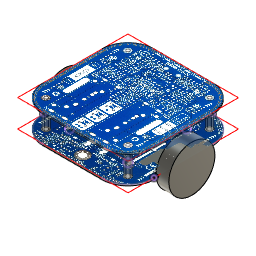
NIBO-Burger_Tuning (Autodesk Fusion 360 design; units mm, degrees)
Autodesk Fusion 360 part; units mm, degrees
sketch "Sketch1" plane through (0, 0, 0) normal (0, 0, 1) x (1, 0, 0) in component "Nibo Burger PCB Bottom"
  line L0 (25.4, 0) -> (82.6, 0)
  line L1 (108, 25.4) -> (108, 82.6)
  line L2 (82.6, 108) -> (25.4, 108)
  line L3 (0, 82.6) -> (0, 25.4)
  arc A0 (25.4, 108) -> (0, 82.6) centre (25.4, 82.6) ccw
  arc A1 (108, 82.6) -> (82.6, 108) centre (82.6, 82.6) ccw
  arc A2 (82.6, 0) -> (108, 25.4) centre (82.6, 25.4) ccw
  arc A3 (0, 25.4) -> (25.4, 0) centre (25.4, 25.4) ccw
  point P0 (108, 0)
  point P1 (0, 108)
  dimension "d1" = 108
  dimension "d2" = 108
  dimension "d5" = 25.4
  constraint horizontal L0
  constraint vertical L1
  constraint horizontal L2
  constraint vertical L3
  constraint coincident P1 L3
  constraint coincident P1 L2
  constraint tangent L3 A0
  constraint tangent L2 A0
  constraint tangent L2 A1
  constraint tangent L1 A1
  constraint equal A0 A1
  constraint coincident P0 L1
  constraint coincident P0 L0
  constraint tangent L1 A2
  constraint tangent L0 A2
  constraint equal A0 A2
  constraint coincident origin L0
  constraint coincident origin L3
  constraint tangent L0 A3
  constraint tangent L3 A3
  constraint equal A0 A3
  measures "d1" distance of origin P0
  measures "d2" distance of origin P1
  measures "d5" radius of A0
extrude "Extrude1" add sketch "Sketch1" along normal blind 1.6 makes body 1 in component "Nibo Burger PCB Bottom"
sketch "Sketch2" plane through (0, 0, 1.6) normal (0, 0, 1) x (-1, 0, 0)
  line L0 (0, -82.6) -> (0, -25.4)
  line L1 (-25.4, 0) -> (-82.6, 0)
  line L2 (-108, -25.4) -> (-108, -82.6)
  line L3 (-82.6, -108) -> (-25.4, -108)
  arc A0 (0, -25.4) -> (-25.4, 0) centre (-25.4, -25.4) ccw
  arc A1 (-82.6, 0) -> (-108, -25.4) centre (-82.6, -25.4) ccw
  arc A2 (-108, -82.6) -> (-82.6, -108) centre (-82.6, -82.6) ccw
  arc A3 (-25.4, -108) -> (0, -82.6) centre (-25.4, -82.6) ccw
copy_body "CopyPasteBodies1" bodies 1 makes body 2 in component "Nibo Burger PCB Bottom"
move_body "Move1" bodies 2 to x (1, 0, 0) y (0, 1, 0) z (0, 0, 1) at (0, 0, 26.5) in component "Nibo Burger PCB Bottom"
copy_body "CutPasteBodies1" bodies 2 removing the originals makes body 3 in component "Nibo Burger PCB Top"
sketch "Sketch1 (2)" plane through (0, 0, 28.1) normal (0, 0, 1) x (-1, 0, 0) in component "Nibo Burger PCB Top"
  arc A0 (0, -25.4) -> (-25.4, 0) centre (-25.4, -25.4) ccw
  line L0 (-25.4, 0) -> (-82.6, 0)
  arc A1 (-82.6, 0) -> (-108, -25.4) centre (-82.6, -25.4) ccw
  line L1 (-108, -25.4) -> (-108, -82.6)
  arc A2 (-108, -82.6) -> (-82.6, -108) centre (-82.6, -82.6) ccw
  line L2 (-82.6, -108) -> (-25.4, -108)
  arc A3 (-25.4, -108) -> (0, -82.6) centre (-25.4, -82.6) ccw
  line L3 (0, -82.6) -> (0, -25.4)
  line L4 (0, -54) -> (-108, -54)
  line L5 (-94, -14) -> (-14, -14)
  line L6 (-14, -14) -> (-14, -94)
  line L7 (-14, -94) -> (-94, -94)
  line L8 (-94, -94) -> (-94, -14)
  line L9 (-94, -14) -> (-14, -94) construction
  line L10 (-14, -14) -> (-94, -94) construction
  point P0 (-54, -54)
  dimension "d7" = 80
  dimension "d8" = 80
  constraint midpoint L3 L4.start
  constraint midpoint L1 L4.end
  constraint horizontal L5
  constraint perpendicular L5 L6
  constraint parallel L5 L7
  constraint parallel L6 L8
  constraint coincident L9 P0
  constraint coincident L10 P0
  constraint midpoint L4 P0
  measures "d7" distance of L6.end L7.end
  measures "d8" distance of L5.end L6.end
hole "Hole1" at (14, 94, 28.1) at (94, 94, 28.1) at (14, 14, 28.1) at (94, 14, 28.1) direction (0, 0, -1) diameter 3.3 depth 30 tip angle 118 bodies 1 in component "Nibo Burger PCB Bottom"
hole "Hole1'" at (14, 94, 28.1) at (94, 94, 28.1) at (14, 14, 28.1) at (94, 14, 28.1) direction (0, 0, -1) diameter 3.3 depth 30 tip angle 118 bodies 3 in component "Nibo Burger PCB Top"
sketch "Sketch2 (2)" plane through (0, 0, 1.6) normal (0, 0, 1) x (-1, 0, 0) in component "Nibo Burger PCB Bottom"
  line L0 (-91.2116, -14.7471) -> (-91.9588, -11.9588)
  line L1 (-91.9588, -11.9588) -> (-94.7471, -11.2116)
  line L2 (-94.7471, -11.2116) -> (-96.7884, -13.2529)
  line L3 (-96.7884, -13.2529) -> (-96.0412, -16.0412)
  line L4 (-96.0412, -16.0412) -> (-93.2529, -16.7884)
  line L5 (-93.2529, -16.7884) -> (-91.2116, -14.7471)
  line L6 (-11.1966, -14.6888) -> (-12.0018, -11.9166)
  line L7 (-12.0018, -11.9166) -> (-14.8052, -11.2278)
  line L8 (-14.8052, -11.2278) -> (-16.8034, -13.3112)
  line L9 (-16.8034, -13.3112) -> (-15.9982, -16.0834)
  line L10 (-15.9982, -16.0834) -> (-13.1948, -16.7722)
  line L11 (-13.1948, -16.7722) -> (-11.1966, -14.6888)
  line L12 (-16.5376, -92.6238) -> (-16.4606, -95.5095)
  line L13 (-16.4606, -95.5095) -> (-13.9231, -96.8857)
  line L14 (-13.9231, -96.8857) -> (-11.4624, -95.3762)
  line L15 (-11.4624, -95.3762) -> (-11.5394, -92.4905)
  line L16 (-11.5394, -92.4905) -> (-14.0769, -91.1143)
  line L17 (-14.0769, -91.1143) -> (-16.5376, -92.6238)
  line L18 (-96.6547, -92.866) -> (-96.3094, -95.7321)
  line L19 (-96.3094, -95.7321) -> (-93.6547, -96.866)
  line L20 (-93.6547, -96.866) -> (-91.3453, -95.134)
  line L21 (-91.3453, -95.134) -> (-91.6906, -92.268)
  line L22 (-91.6906, -92.268) -> (-94.3453, -91.134)
  line L23 (-94.3453, -91.134) -> (-96.6547, -92.866)
  point P0 (-94, -14)
  point P1 (-14, -14)
  point P2 (-14, -94)
  point P3 (-94, -94)
  dimension "d15" = 2.5
  dimension "d16" = 2.5
  dimension "d17" = 2.5
  dimension "d18" = 2.5
  measures "d15" distance of P0 L5
  measures "d16" distance of P1 L11
  measures "d17" distance of P2 L17
  measures "d18" distance of P3 L23
extrude "Extrude2" add sketch "Sketch2 (2)" along normal blind 25 separate body makes body 4 at (14.8972, 91.6174, 9.9333) makes body 5 at (91.4607, 13.8177, 9.9333) makes body 6 at (16.535, 14.2353, 9.9333) makes body 7 at (91.4604, 94.1786, 9.9333) in component "Nibo Burger PCB Bottom"
sketch "Sketch3" plane through (0, 0, 1.6) normal (0, 0, 1) x (-1, 0, 0) in component "Nibo Burger PCB Bottom"
  line L0 (0, 0) -> (0, -54)
  line L1 (0, -54) -> (-108, -54)
  line L2 (-5.5, -78) -> (5.5, -78)
  line L3 (5.5, -78) -> (5.5, -30)
  line L4 (5.5, -30) -> (-5.5, -30)
  line L5 (-5.5, -30) -> (-5.5, -78)
  line L6 (-5.5, -78) -> (5.5, -30) construction
  line L7 (5.5, -78) -> (-5.5, -30) construction
  line L8 (-102.5, -78) -> (-113.5, -78)
  line L9 (-113.5, -78) -> (-113.5, -30)
  line L10 (-113.5, -30) -> (-102.5, -30)
  line L11 (-102.5, -30) -> (-102.5, -78)
  line L12 (-102.5, -78) -> (-113.5, -30) construction
  line L13 (-113.5, -78) -> (-102.5, -30) construction
  point P0 (0, -54)
  point P1 (-108, -54)
  dimension "d22" = 54
  dimension "d23" = 108
  dimension "d24" = 11
  dimension "d25" = 48
  dimension "d26" = 11
  dimension "d27" = 48
  constraint coincident L0.start origin
  constraint vertical L0
  constraint perpendicular L0 L1
  constraint horizontal L2
  constraint perpendicular L2 L3
  constraint parallel L2 L4
  constraint parallel L3 L5
  constraint coincident L6 P0
  constraint coincident L7 P0
  constraint coincident P0 L0.end
  constraint horizontal L8
  constraint perpendicular L8 L9
  constraint parallel L8 L10
  constraint parallel L9 L11
  constraint coincident L12 P1
  constraint coincident L13 P1
  constraint coincident P1 L1.end
  measures "d22" distance of L0.start P0
  measures "d23" distance of P0 P1
  measures "d24" distance of L3.end L4.end
  measures "d25" distance of L2.end L3.end
  measures "d26" distance of L9.end L10.end
  measures "d27" distance of L8.end L9.end
extrude "Extrude3" cut sketch "Sketch3" against normal blind 10 bodies 1 in component "Nibo Burger PCB Bottom"
sketch "Sketch4" plane through (0, 0, 0) normal (-1, 0, 0) x (0, -1, 0) in component "Nibo Burger PCB Bottom"
  line L0 (-78, 0) -> (-78, 1.6)
  line L1 (-78, 1.6) -> (-82.6, 1.6)
  line L2 (-82.6, 1.6) -> (-82.6, 0)
  line L3 (-82.6, 0) -> (-78, 0)
  line L4 (-78, 1.6) -> (-30, 1.6)
  circle A0 centre (-54, -0.7) radius 22.5
  circle A1 through (-31.5, -0.7, -108) (-65.25, 18.7856, -108) (-65.25, -20.1856, -108)
  dimension "d30" = 45
  dimension "d31" = 45
  constraint coincident L0.end L1.start
  constraint perpendicular L0 L4
  measures "d30" diameter of A0
extrude "Extrude4" add sketch "Sketch4" along normal blind 8.5 separate body contours L4 A0 | L4 A0 makes body 8 in component "Nibo Burger PCB Bottom"
extrude "Extrude5" add sketch "Sketch4" against normal blind 8.5 separate body contours A1 in plane through (108, 0, 0) normal (-1, 0, 0) makes body 9 in component "Nibo Burger PCB Bottom"
extrude "Extrude6" add sketch "Sketch4" against normal blind 4 contours L4 A0 | L4 A0 bodies 8 in component "Nibo Burger PCB Bottom"
extrude "Extrude7" add sketch "Sketch4" along normal blind 4 contours A1 in plane through (108, 0, 0) normal (-1, 0, 0) bodies 9 in component "Nibo Burger PCB Bottom"
copy_body "CutPasteBodies1'" bodies 9 removing the originals makes body 10 in component "Nibo Burger Wheels"
copy_body "CutPasteBodies2" bodies 8 removing the originals makes body 11 in component "Nibo Burger Wheels"
copy_body "CutPasteBodies1''" bodies 4 removing the originals makes body 12 in component "Nibo Burger PCB Standoff"
copy_body "CutPasteBodies2'" bodies 5 removing the originals makes body 13 in component "Nibo Burger PCB Standoff"
copy_body "CutPasteBodies3" bodies 6 removing the originals makes body 14 in component "Nibo Burger PCB Standoff"
copy_body "CutPasteBodies4" bodies 7 removing the originals makes body 15 in component "Nibo Burger PCB Standoff"
component "Nibo Burger PCB Bottom" placed x (1, 0, 0) y (0, 1, 0) z (0, 0, 1) at (0, 0, 0)
component "Nibo Burger PCB Top" placed x (1, 0, 0) y (0, 1, 0) z (0, 0, 1) at (0, 0, 0.1)
component "Nibo Burger Wheels" placed x (1, 0, 0) y (0, 1, 0) z (0, 0, 1) at (0, 0, 0)
component "Nibo Burger PCB Standoff" placed x (1, 0, 0) y (0, 1, 0) z (0, 0, 1) at (0, 0, 0)
named bodies: "PCB$", "PCB", "Wheel right", "Wheel left", "Standoff front left", "Standoff back right", "Standoff back left", "Standoff front right"
